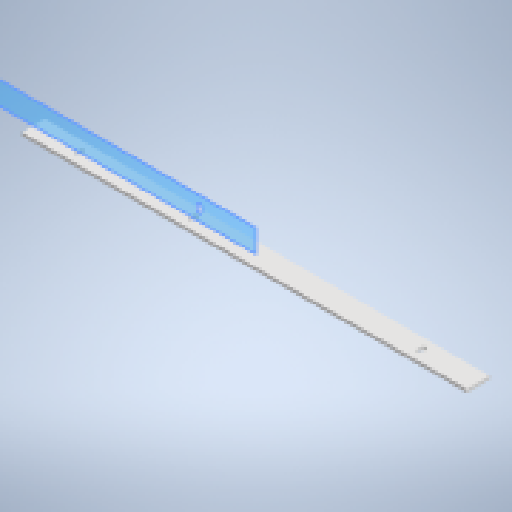
# Autodesk Inventor part: 발받침대좌,우
Saved by Autodesk Inventor 2024 (Build 280153000, 153)
## iProperties
Created: 2024-04-09
Part Number: 발받침대좌,우
Material: 일반
Document SubType Name: Modeling
Designer: ckhye
Density: 1 g/cm^3
Appearance: 기본값
Author: ckhye
Autodesk Inventor part; units mm, degrees
ref_plane "YZ Plane" through (0, 0, 0) normal (1, 0, 0) x (0, 1, 0)
ref_plane "XZ Plane" through (0, 0, 0) normal (0, 1, 0) x (-1, 0, 0)
ref_plane "XY Plane" through (0, 0, 0) normal (0, 0, 1) x (1, 0, 0)
sketch "스케치1" plane through (0, 0, 0) normal (0, 1, 0) x (-1, 0, 0)
  line L0 (195, 10) -> (-195, 10)
  line L1 (-195, 10) -> (-195, -10)
  line L2 (-195, -10) -> (195, -10)
  line L3 (195, -10) -> (195, 10)
  line L4 (195, 10) -> (-195, -10) construction
  line L5 (-195, 10) -> (195, -10) construction
  point P0 (0, 0)
  dimension "d0" = 390
  dimension "d1" = 20
  constraints: 12 end point, 2 midpoint, 2 parallel, 1 horizontal, 1 perpendicular
  measures "d0" distance of L2.end L1.end
  measures "d1" distance between parallel lines of L2 L0
extrude "돌출1" add sketch "스케치1" along normal blind 3
sketch "스케치3" plane through (0, 3, 0) normal (0, 1, 0) x (1, 0, 0)
  line L0 (-155, 2) -> (-155, -2) construction
  line L1 (-157, 2) -> (-157, -2)
  line L2 (-153, -2) -> (-153, 2)
  arc A0 (-153, 2) -> (-157, 2) centre (-155, 2) ccw
  arc A1 (-157, -2) -> (-153, -2) centre (-155, -2) ccw
  line L3 (-195, 10) -> (-195, -10) projected
  line L4 (-55, 2) -> (-55, -2) construction
  line L5 (-57, 2) -> (-57, -2)
  line L6 (-53, -2) -> (-53, 2)
  arc A2 (-53, 2) -> (-57, 2) centre (-55, 2) ccw
  arc A3 (-57, -2) -> (-53, -2) centre (-55, -2) ccw
  line L7 (145, 2) -> (145, -2) construction
  line L8 (143, 2) -> (143, -2)
  line L9 (147, -2) -> (147, 2)
  arc A4 (147, 2) -> (143, 2) centre (145, 2) ccw
  arc A5 (143, -2) -> (147, -2) centre (145, -2) ccw
  line L10 (195, -10) -> (195, 10) projected
  point P0 (0, 0)
  point P1 (-155, 0)
  point P2 (-195, 0)
  point P3 (-195, 0)
  point P4 (-55, 0)
  point P5 (145, 0)
  point P6 (195, 0)
  point P7 (195, 0)
  dimension "d14" = 4
  dimension "d15" = 4
  dimension "d16" = 0
  dimension "d17" = 40
  dimension "d18" = 4
  dimension "d19" = 4
  dimension "d20" = 100
  dimension "d21" = 0
  dimension "d22" = 4
  dimension "d23" = 4
  dimension "d24" = 0
  dimension "d25" = 50
  constraints: 24 end point, 12 point on circle, 12 tangent, 7 midpoint, 6 centre point, 3 parallel, 3 vertical
  measures "d14" distance of L0.start L0.end
  measures "d15" diameter of A1
  measures "d16" vertical distance of point (-195, 0) point (-155, 0)
  measures "d17" distance of point (-195, 0) point (-155, 0)
  measures "d18" distance of L4.start L4.end
  measures "d19" diameter of A3
  measures "d20" distance of point (-155, 0) point (-55, 0)
  measures "d21" vertical distance of point (-155, 0) point (-55, 0)
  measures "d22" distance of L7.start L7.end
  measures "d23" diameter of A5
  measures "d24" vertical distance of point (195, 0) point (145, 0)
  measures "d25" distance of point (145, 0) point (195, 0)
extrude "돌출2" cut sketch "스케치3" against normal blind 10
